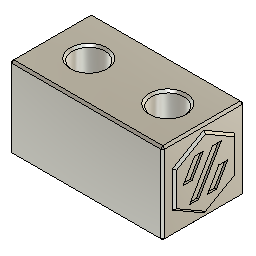
Fystec M5 Insert Nut Block v4 (Autodesk Fusion 360 design; units mm, degrees)
Autodesk Fusion 360 part; units mm, degrees
sketch "Sketch1" plane through (0, 0, 0) normal (0, 0, 1) x (1, 0, 0)
  line L0 (0, 0) -> (30, 0)
  line L1 (30, 0) -> (30, 16)
  line L2 (30, 16) -> (0, 16)
  line L3 (0, 16) -> (0, 0)
  dimension "d1" = 30
  dimension "d2" = 16
  constraint horizontal L0
  constraint vertical L1
  constraint horizontal L2
  constraint vertical L3
  constraint coincident L0.start L3.end
  measures "d1" distance of L0.start L0.end
  measures "d2" distance of L0.start L2.end
extrude "Extrude1" add sketch "Sketch1" along normal blind 16
sketch "Sketch2" plane through (0, 0, 16) normal (0, 0, 1) x (-1, 0, 0)
  line L0 (0, -16) -> (0, 0)
  line L1 (0, 0) -> (-30, 0)
  line L2 (-30, 0) -> (-30, -16)
  line L3 (-30, -16) -> (0, -16)
  line L4 (0, -8) -> (-30, -8) construction
  line L5 (-7.5, -16) -> (-7.5, 0) construction
  line L6 (-23, -16) -> (-23, 0) construction
  circle A0 centre (-7.5, -8) radius 3.2
  circle A1 centre (-23, -8) radius 3.2
  dimension "d5" = 7.5
  dimension "d6" = 15.5
  dimension "d7" = 6.4
  dimension "d8" = 6.4
  constraint midpoint L0 L4.start
  constraint midpoint L2 L4.end
  constraint coincident L3 L5.start
  constraint coincident L1 L5.end
  constraint perpendicular L1 L5
  constraint coincident L3 L6.start
  constraint coincident L1 L6.end
  constraint perpendicular L1 L6
  constraint midpoint L5 A0.centre
  constraint midpoint L6 A1.centre
  measures "d5" distance of L0 L5
  measures "d6" distance of L5 L6
  measures "d7" diameter of A0
  measures "d8" diameter of A1
extrude "Extrude2" cut sketch "Sketch2" against normal blind 6 contours A0 | A1
sketch "Sketch3" plane through (0, 0, 0) normal (0, 0, -1) x (1, 0, 0)
  line L0 (0, 0) -> (0, -16)
  line L1 (0, -16) -> (30, -16)
  line L2 (30, -16) -> (30, 0)
  line L3 (30, 0) -> (0, 0)
  circle A0 centre (7.5, -8) radius 3.2
  circle A1 centre (23, -8) radius 3.2
extrude "Extrude3" cut sketch "Sketch3" against normal blind 6 contours A0 | A1
sketch "Sketch4" plane through (30, 0, 0) normal (1, 0, 0) x (0, 1, 0)
  line L0 (0, 0) -> (16, 0)
  line L1 (16, 0) -> (16, 16)
  line L2 (16, 16) -> (0, 16)
  line L3 (0, 16) -> (0, 0)
  line L4 (7.6049, 11.8719) -> (5.3694, 8)
  line L5 (12.3843, 8) -> (10.1488, 4.1281)
  line L6 (1.925, 11.5074) -> (8, 15.0148)
  line L7 (5.8512, 11.8719) -> (7.6049, 11.8719)
  line L8 (3.6157, 8) -> (5.8512, 11.8719)
  line L9 (9.3586, 11.8719) -> (4.8877, 4.1281)
  line L10 (14.075, 11.5074) -> (14.075, 4.4926)
  line L11 (6.6414, 4.1281) -> (11.1123, 11.8719)
  line L12 (10.6306, 8) -> (12.3843, 8)
  line L13 (8, 15.0148) -> (14.075, 11.5074)
  line L14 (8, 0.9852) -> (1.925, 4.4926)
  line L15 (1.925, 4.4926) -> (1.925, 11.5074)
  line L16 (8.3951, 4.1281) -> (10.6306, 8)
  line L17 (5.3694, 8) -> (3.6157, 8)
  line L18 (4.8877, 4.1281) -> (6.6414, 4.1281)
  line L19 (11.1123, 11.8719) -> (9.3586, 11.8719)
  line L20 (10.1488, 4.1281) -> (8.3951, 4.1281)
  line L21 (14.075, 4.4926) -> (8, 0.9852)
  line L22 (7.0257, 8) -> (8.9743, 8) construction
  line L23 (0, 8) -> (16, 8) construction
  line L24 (8, 16) -> (8, 0) construction
  point P0 (8, 8)
  point P1 (8, 8)
  constraint horizontal L22
  constraint midpoint L3 L23.start
  constraint midpoint L1 L23.end
  constraint midpoint L2 L24.start
  constraint midpoint L0 L24.end
  constraint midpoint L22 P1
  constraint midpoint L24 P1
extrude "Extrude4" add sketch "Sketch4" along normal blind 0.4 contours L6 L10 L13 L14 L15 L21
chamfer "Chamfer1" distance 0.4 angle 45 12 edges at (15, 0, 16) (30, 8, 16) (30, 0, 8) (30, 16, 8) (15, 16, 16) (0, 8, 16) (0, 16, 8) (15, 16, 0) (15, 0, 0) (0, 8, 0) (0, 0, 8) (30, 8, 0)
chamfer "Chamfer2" distance 0.4 angle 45 6 edges at (30.4, 4.9625, 13.2611) (30.4, 11.0375, 13.2611) (30.4, 1.925, 8) (30.4, 4.9625, 2.7389) (30.4, 11.0375, 2.7389) (30.4, 14.075, 8)
chamfer "Chamfer3" distance 0.4 angle 45 4 edges at (10.4834, 6.8428, 16) (25.9834, 6.8428, 16) (4.5166, 6.8428, 0) (20.0166, 6.8428, 0)
chamfer "Chamfer4" distance 0.6 angle 45 4 edges at (25.9834, 6.8428, 10) (10.4834, 6.8428, 10) (20.0166, 6.8428, 6) (4.5166, 6.8428, 6)
extrude "Extrude7" cut 2 faces at (8.3097, 7.9914, 10) (22.2885, 9.0947, 10) along direction (0, 0, -1) blind 4
